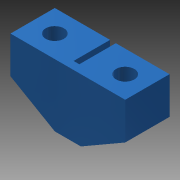
# Autodesk Inventor part: XCarriageBeltClip
Saved by Autodesk Inventor 2015 (Build 190159000, 159)
## iProperties
Created: 2014-12-05
Part Number: XCarriageBeltClip
Material: ABS Plastic
Document SubType Name: Modeling
Designer: Jack
Density: 1.06 g/cm^3
Appearance: Cyan
Author: Jack
Autodesk Inventor part; units mm, degrees
ref_plane "YZ Plane" through (0, 0, 0) normal (1, 0, 0) x (0, 1, 0)
ref_plane "XZ Plane" through (0, 0, 0) normal (0, 1, 0) x (-1, 0, 0)
ref_plane "XY Plane" through (0, 0, 0) normal (0, 0, 1) x (1, 0, 0)
sketch "Sketch1" plane through (0, 0, 0) normal (0, 1, 0) x (-1, 0, 0)
  line L0 (0, 0) -> (0, -7.0925)
  line L1 (0, -7.0925) -> (8.5, -12)
  line L2 (8.5, -12) -> (13.5, -12)
  line L3 (13.5, -12) -> (22, -7.0925)
  line L4 (22, -7.0925) -> (22, 0)
  line L5 (22, 0) -> (0, 0)
  dimension "d0" = 12
  dimension "d1" = 150
  dimension "d2" = 150
  dimension "d3" = 22
  dimension "d4" = 5
  constraints: 12 end point, 2 perpendicular, 1 equal length, 1 parallel, 1 vertical
  measures "d0" distance between parallel lines of L2 L5
  measures "d1" angle of L2 L3
  measures "d2" angle of L2 L1
  measures "d3" distance between parallel lines of L4 L0
  measures "d4" distance of L1.end L2.end
extrude "Extrusion1" add sketch "Sketch1" along normal blind 8.5
sketch "Sketch2" plane through (0, 8.5, 0) normal (0, 1, 0) x (1, 0, 0)
  line L0 (-8.5, 12) -> (-13.5, 12) projected
  line L1 (-22, 7.0925) -> (-22, 0) projected
  line L2 (-22, 0) -> (0, 0) projected
  line L3 (-11.4, 12) -> (-11.4, 0)
  arc A0 (-10.3, 0) -> (-10.3, 1.1) centre (-10.3, 0.55) ccw
  line L4 (-10.6, 1.1) -> (-10.6, 2)
  line L5 (-10.3, 1.1) -> (-10.6, 1.1)
  line L6 (-10.6, 2) -> (-11.4, 2)
  dimension "d7" = 10.6
  dimension "d8" = 1.1
  dimension "d9" = 1.1
  dimension "d10" = 0.55
  dimension "d11" = 0.8
  dimension "d13" = 0.9
  constraints: 8 end point, 4 point on line, 2 horizontal, 2 point on circle, 2 vertical, 1 centre point, 1 tangent
  measures "d7" distance between parallel lines of L1 L3
  measures "d8" diameter of A0
  measures "d9" distance from line of L3 A0.centre
  measures "d10" distance from line of L2 A0.centre
  measures "d11" distance between parallel lines of L3 L4
  measures "d13" distance of L4.start L4.end
extrude "Extrusion2" cut sketch "Sketch2" against normal blind 7
pattern_linear "Rectangular Pattern1" count 6 spacing 2 along (0, 0, -1) of "Extrusion2"
sketch "Sketch3" plane through (-8.5, 0, -12) normal (0, 0, -1) x (-1, 0, 0)
  line L0 (-8.5, 0) -> (0, 0) projected
  line L1 (0, 0) -> (0, 8.5) projected
  line L2 (-8.5, 8.5) -> (0, 8.5) projected
  line L3 (-8.5, 0) -> (-8.5, 8.5) projected
  line L4 (5, 0) -> (13.5, 0) projected
  line L5 (13.5, 0) -> (13.5, 8.5) projected
  line L6 (5, 8.5) -> (13.5, 8.5) projected
  line L7 (5, 0) -> (5, 8.5) projected
  point P0 (-4.25, 4.25)
  point P1 (9.25, 4.25)
  dimension "d19" = 4.25
  dimension "d20" = 4.25
  dimension "d21" = 4.25
  constraints: 1 horizontal alignment
  measures "d19" distance from line of L6 point (9.25, 4.25)
  measures "d20" distance from line of point (-4.25, 4.25) L3
  measures "d21" distance from line of L5 point (9.25, 4.25)
hole "Hole1" at (-4.25, 4.25, -12) at (-17.75, 4.25, -12) direction (0, 0, 1) diameter 3.5 end through all counterbore diameter 8 counterbore depth 5
body "Solid1"
